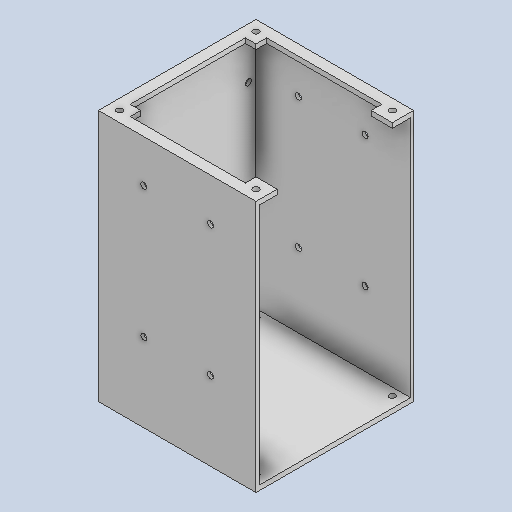
# Autodesk Inventor part: Part15
Saved by Autodesk Inventor 2025 (Build 290162000, 162)
## iProperties
Created: 2025-08-11
Part Number: Part15
Material: Generic
Document SubType Name: Modeling
Designer: Pravoslav
Density: 1 g/cm^3
Appearance: Default
Author: Pravoslav
Autodesk Inventor part; units mm, degrees
ref_plane "YZ Plane" through (0, 0, 0) normal (1, 0, 0) x (0, 1, 0)
ref_plane "XZ Plane" through (0, 0, 0) normal (0, 1, 0) x (-1, 0, 0)
ref_plane "XY Plane" through (0, 0, 0) normal (0, 0, 1) x (1, 0, 0)
sketch "Sketch1" plane through (0, 0, 0) normal (0, 1, 0) x (-1, 0, 0)
  line L0 (65, 65) -> (-65, 65)
  line L1 (-65, 65) -> (-65, -65)
  line L2 (-65, -65) -> (65, -65)
  line L3 (65, -65) -> (65, 65)
  line L4 (65, 65) -> (-65, -65) construction
  line L5 (-65, 65) -> (65, -65) construction
  circle A0 centre (-56.25, 56.25) radius 2.5
  line L6 (0, 15.2849) -> (0, -21.0051)
  line L7 (0, -21.0051) -> (-20.003, 0)
  line L8 (-20.003, 0) -> (15.941, 0)
  circle A1 centre (56.25, 56.25) radius 2.5
  circle A2 centre (-56.25, -56.25) radius 2.5
  circle A3 centre (56.25, -56.25) radius 2.5
  point P0 (0, 0)
  point P1 (0, 0)
  dimension "d0" = 130
  dimension "d1" = 130
  dimension "d2" = 5
  dimension "d3" = 8.75
  constraints: 18 end point, 4 centre point, 3 symmetric about line, 2 midpoint, 2 parallel, 2 perpendicular, 1 horizontal, 1 point on line, 1 vertical, 3 other
  measures "d0" distance of L2.end L1.end
  measures "d1" distance of L1.end L0.end
  measures "d2" diameter of A0
  measures "d3" distance from line of L0 A0.centre
extrude "Extrusion1" add sketch "Sketch1" along normal blind 4 contours L3 L2 L1 L0 | L6 L7 L8
sketch "Sketch2" plane through (0, 4, 0) normal (0, 1, 0) x (1, 0, 0)
  line L0 (-62.5, -62.5) -> (62.5, -62.5)
  line L1 (62.5, -62.5) -> (62.5, 62.5)
  line L2 (62.5, 62.5) -> (-62.5, 62.5)
  line L3 (-62.5, 62.5) -> (-62.5, -62.5)
  line L4 (-62.5, -62.5) -> (62.5, 62.5) construction
  line L5 (62.5, -62.5) -> (-62.5, 62.5) construction
  line L6 (-65, 65) -> (-65, -65) projected
  line L7 (65, 65) -> (-65, 65) projected
  line L8 (-65, -65) -> (65, -65)
  line L9 (65, -65) -> (65, 65)
  line L10 (65, 65) -> (-65, 65)
  line L11 (-65, 65) -> (-65, -65)
  line L12 (-65, -65) -> (65, 65) construction
  line L13 (65, -65) -> (-65, 65) construction
  line L14 (62.5, -62.5) -> (65, -62.5)
  line L15 (62.5, 62.5) -> (65, 62.5)
  point P0 (0, 0)
  dimension "d6" = 2.5
  dimension "d7" = 2.5
  constraints: 28 end point, 4 midpoint, 4 parallel, 3 perpendicular, 3 point on line, 2 horizontal
  measures "d6" distance between parallel lines of L6 L3
  measures "d7" distance between parallel lines of L7 L2
extrude "Extrusion2" add sketch "Sketch2" along normal blind 204 contours L0 L14 L9 L8 L6 L7 L15 L2 L3
sketch "Sketch3" plane through (0, 208, 0) normal (0, 1, 0) x (1, 0, 0)
  line L0 (-65, 65) -> (-65, -65) projected
  line L1 (-65, -65) -> (-47.5, -65)
  line L2 (-47.5, -65) -> (-47.5, -47.5)
  line L3 (-47.5, -47.5) -> (-65, -47.5)
  line L4 (-65, -47.5) -> (-65, -65)
  line L5 (-65, 65) -> (-47.5, 65)
  line L6 (-47.5, 65) -> (-47.5, 47.5)
  line L7 (-47.5, 47.5) -> (-65, 47.5)
  line L8 (-65, 47.5) -> (-65, 65)
  line L9 (-65, -65) -> (65, -65) projected
  line L10 (65, -65) -> (47.5, -65)
  line L11 (47.5, -65) -> (47.5, -47.5)
  line L12 (47.5, -47.5) -> (65, -47.5)
  line L13 (65, -47.5) -> (65, -65)
  line L14 (65, 65) -> (-65, 65) projected
  line L15 (65, 65) -> (47.5, 65)
  line L16 (47.5, 65) -> (47.5, 47.5)
  line L17 (47.5, 47.5) -> (65, 47.5)
  line L18 (65, 47.5) -> (65, 65)
  circle A0 centre (56.25, -56.25) radius 2.5
  circle A1 centre (56.25, 56.25) radius 2.5 projected
  circle A2 centre (56.25, 56.25) radius 2.5
  circle A3 centre (-56.25, 56.25) radius 2.5
  circle A4 centre (-56.25, -56.25) radius 2.5 projected
  circle A5 centre (-56.25, -56.25) radius 2.5
  line L19 (-47.5, -56.25) -> (47.5, -56.25)
  line L20 (-56.25, -47.5) -> (-56.25, 47.5)
  line L21 (-47.5, 56.25) -> (47.5, 56.25)
  point P0 (0, 0)
  point P1 (56.25, -65)
  dimension "d10" = 17.5
  dimension "d11" = 17.5
  dimension "d12" = 17.5
  dimension "d13" = 17.5
  dimension "d14" = 17.5
  dimension "d15" = 17.5
  dimension "d16" = 17.5
  dimension "d17" = 17.5
  dimension "d18" = 5
  dimension "d19" = 5
  dimension "d20" = 5
  dimension "d21" = 5
  constraints: 38 end point, 8 parallel, 7 midpoint, 4 centre point, 4 horizontal, 4 perpendicular, 2 coincident
  measures "d10" distance of L3.end L2.end
  measures "d11" distance between parallel lines of L1 L3
  measures "d12" distance of L6.end L7.end
  measures "d13" distance of L5.end L6.end
  measures "d14" distance of L11.end L12.end
  measures "d15" distance from line of point (56.25, -65) L12
  measures "d16" distance of L17.end L16.end
  measures "d17" distance of L16.end L15.end
  measures "d18" diameter of A0
  measures "d19" diameter of A2
  measures "d20" diameter of A3
  measures "d21" diameter of A5
extrude "Extrusion3" add sketch "Sketch3" against normal blind 4
sketch "Sketch4" plane through (-65, 0, -65) normal (-1, 0, 0) x (0, 0, 1)
  circle A0 centre (8.75, 168.75) radius 2.5
  circle A1 centre (121.25, 168.75) radius 2.5
  line L0 (0, 208) -> (130, 208) projected
  line L1 (0, 0) -> (0, 208) projected
  line L2 (130, 0) -> (130, 208) projected
  point P0 (65, 0)
  dimension "d24" = 5
  dimension "d25" = 5
  dimension "d26" = 39.25
  dimension "d27" = 39.25
  dimension "d28" = 8.75
  dimension "d29" = 8.75
  constraints: 2 centre point
  measures "d24" diameter of A0
  measures "d25" diameter of A1
  measures "d26" distance from line of A0.centre L0
  measures "d27" distance from line of L0 A1.centre
  measures "d28" distance from line of L1 A0.centre
  measures "d29" distance from line of L2 A1.centre
extrude "Extrusion4" cut sketch "Sketch4" against normal through all
sketch "Sketch7" plane through (-65, 0, 65) normal (0, 0, 1) x (1, 0, 0)
  circle A0 centre (37.5, 173) radius 2.5
  circle A1 centre (92.5, 173) radius 2.5
  circle A2 centre (37.5, 65) radius 2.5
  circle A3 centre (92.5, 65) radius 2.5
  line L0 (0, 208) -> (130, 208) projected
  line L1 (130, 0) -> (130, 208) projected
  line L2 (0, 0) -> (130, 0) projected
  point P0 (65, 0)
  dimension "d47" = 5
  dimension "d48" = 5
  dimension "d49" = 5
  dimension "d50" = 5
  dimension "d51" = 55
  dimension "d52" = 55
  dimension "d53" = 0
  dimension "d54" = 35
  dimension "d55" = 0
  dimension "d56" = 37.5
  dimension "d57" = 37.5
  dimension "d58" = 65
  constraints: 4 centre point
  measures "d47" diameter of A0
  measures "d48" diameter of A1
  measures "d49" diameter of A2
  measures "d50" diameter of A3
  measures "d51" distance of A3.centre A2.centre
  measures "d52" distance of A1.centre A0.centre
  measures "d53" vertical distance of A2.centre A3.centre
  measures "d54" distance from line of L0 A1.centre
  measures "d55" vertical distance of A1.centre A0.centre
  measures "d56" distance from line of L1 A1.centre
  measures "d57" distance from line of L1 A3.centre
  measures "d58" distance from line of L2 A2.centre
sketch "Sketch5" plane through (65, 0, -65) normal (0, 0, -1) x (-1, 0, 0)
  circle A0 centre (37.5, 173) radius 2.5
  circle A1 centre (92.5, 173) radius 2.5
  circle A2 centre (37.5, 65) radius 2.5
  circle A3 centre (92.5, 65) radius 2.5
  line L0 (130, 0) -> (130, 208) projected
  line L1 (0, 208) -> (130, 208) projected
  line L2 (0, 0) -> (130, 0) projected
  point P0 (65, 0)
  dimension "d32" = 5
  dimension "d33" = 5
  dimension "d34" = 5
  dimension "d35" = 5
  dimension "d36" = 55
  dimension "d37" = 55
  dimension "d38" = 0
  dimension "d39" = 37.5
  dimension "d40" = 37.5
  dimension "d41" = 35
  dimension "d42" = 65
  dimension "d43" = 35
  constraints: 4 centre point
  measures "d32" diameter of A0
  measures "d33" diameter of A1
  measures "d34" diameter of A2
  measures "d35" diameter of A3
  measures "d36" distance of A1.centre A0.centre
  measures "d37" distance of A3.centre A2.centre
  measures "d38" vertical distance of A2.centre A3.centre
  measures "d39" distance from line of L0 A1.centre
  measures "d40" distance from line of L0 A3.centre
  measures "d41" distance from line of L1 A0.centre
  measures "d42" distance from line of L2 A2.centre
  measures "d43" distance from line of L1 A1.centre
extrude "Extrusion5" cut sketch "Sketch5" against normal blind 10
sketch "Sketch6" plane through (65, 0, -65) normal (0, 0, -1) x (-1, 0, 0)
  point P0 (65, 0)
mirror "Mirror1" about plane through (0, 0, 0) normal (0, 0, 1) of "Extrusion5"
body "Solid1"
